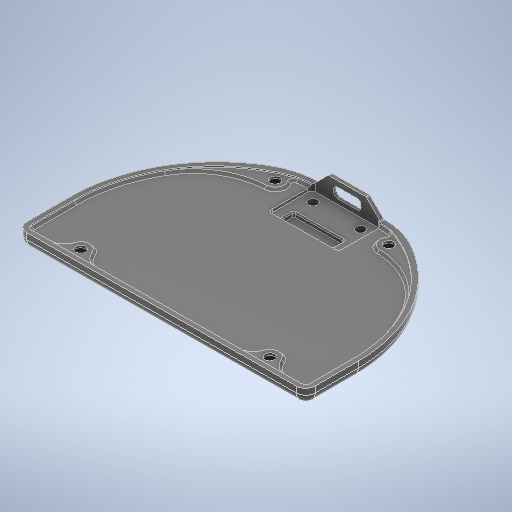
# Autodesk Inventor part: Bottom
Saved by Autodesk Inventor 2025.3 (Build 293356030, 356C)
## iProperties
Created: 2024-12-25
Part Number: Bottom
Material: Acetal Resin, Black
Document SubType Name: Modeling
Designer: tvoko
Density: 1.425 g/cm^3
Appearance: Smooth - Black
Author: tvoko
Autodesk Inventor part; units mm, degrees
ref_plane "YZ Plane" through (0, 0, 0) normal (1, 0, 0) x (0, 1, 0)
ref_plane "XZ Plane" through (0, 0, 0) normal (0, 1, 0) x (-1, 0, 0)
ref_plane "XY Plane" through (0, 0, 0) normal (0, 0, 1) x (1, 0, 0)
ref_plane "Work Plane1" through (11.8275, -6.9783, -10.6662) normal (0.0061942, -0.9999808, -0.0000034) x (0.9999802, 0.0061942, -0.0010922)
sketch "Sketch1" plane through (11.8275, -6.9783, -10.6662) normal (0.0061942, -0.9999808, -0.0000034) x (0.9999802, 0.0061942, -0.0010922)
  line L0 (-55.0975, -59.86) -> (-32.8725, -59.86)
  line L1 (-1.1225, 0.465) -> (-86.8475, 0.465)
  line L2 (-32.8725, -61.4475) -> (-55.0975, -61.4475)
  line L3 (-86.8475, 2.0525) -> (-1.1225, 2.0525)
  circle A0 centre (-24.935, -55.287) radius 1.6
  circle A1 centre (-63.035, -55.287) radius 1.6
  circle A2 centre (-75.735, -2.535) radius 1.6
  circle A3 centre (-12.235, -2.535) radius 1.6
  line L4 (-7.8704, 0.465) -> (-16.5997, 0.465)
  line L5 (-71.3704, 0.465) -> (-80.0997, 0.465)
  line L6 (-55.2619, -59.8595) -> (-55.2619, -61.447) projected
  arc A4 (-59.548, -59.4404) -> (-55.2619, -59.8595) centre (-55.0975, -36.0475) ccw projected
  arc A5 (-60.5607, -56.9833) -> (-59.548, -59.4404) centre (-59.2513, -57.8809) ccw projected
  arc A6 (-60.5607, -56.9833) -> (-62.9204, -52.2892) centre (-63.035, -55.287) ccw projected
  arc A7 (-84.3659, -39.412) -> (-62.9204, -52.2892) centre (-61.9279, -26.3401) ccw projected
  arc A8 (-90.8163, -15.5257) -> (-84.3659, -39.412) centre (-43.3648, -15.5257) ccw projected
  line L7 (-90.8163, -15.5257) -> (-90.8163, -1.1225) projected
  arc A9 (-89.2288, 0.465) -> (-90.8163, -1.1225) centre (-89.2288, -1.1225) ccw projected
  line L8 (-89.2288, 0.465) -> (-84.4643, 0.465) projected
  arc A10 (-78.5359, -3.6099) -> (-84.4643, 0.465) centre (-84.4643, -5.885) ccw projected
  arc A11 (-78.5359, -3.6099) -> (-72.9342, -3.6099) centre (-75.735, -2.535) ccw projected
  arc A12 (-67.0058, 0.465) -> (-72.9342, -3.6099) centre (-67.0058, -5.885) ccw projected
  line L9 (-67.0058, 0.465) -> (-20.9643, 0.465) projected
  arc A13 (-15.0359, -3.6099) -> (-20.9643, 0.465) centre (-20.9643, -5.885) ccw projected
  arc A14 (-15.0359, -3.6099) -> (-9.4342, -3.6099) centre (-12.235, -2.535) ccw projected
  arc A15 (-3.5058, 0.465) -> (-9.4342, -3.6099) centre (-3.5058, -5.885) ccw projected
  line L10 (-3.5058, 0.465) -> (1.2587, 0.465) projected
  arc A16 (2.8462, -1.1225) -> (1.2587, 0.465) centre (1.2587, -1.1225) ccw projected
  line L11 (2.8462, -1.1225) -> (2.8462, -15.5257) projected
  arc A17 (-3.6042, -39.412) -> (2.8462, -15.5257) centre (-44.6053, -15.5257) ccw projected
  arc A18 (-25.0497, -52.2892) -> (-3.6042, -39.412) centre (-26.0422, -26.3401) ccw projected
  arc A19 (-25.0497, -52.2892) -> (-27.4094, -56.9833) centre (-24.935, -55.287) ccw projected
  arc A20 (-28.4221, -59.4404) -> (-27.4094, -56.9833) centre (-28.7188, -57.8809) ccw projected
  arc A21 (-32.7081, -59.8595) -> (-28.4221, -59.4404) centre (-32.8725, -36.0475) ccw projected
  line L12 (-32.7081, -61.447) -> (-32.7081, -59.8595) projected
  arc A22 (-32.7081, -61.447) -> (-20.2658, -58.0981) centre (-32.8725, -36.0475) ccw projected
  arc A23 (-20.2658, -58.0981) -> (4.4337, -15.5257) centre (-44.6053, -15.5257) ccw projected
  line L13 (4.4337, -1.1225) -> (4.4337, -15.5257) projected
  arc A24 (4.4337, -1.1225) -> (1.2587, 2.0525) centre (1.2587, -1.1225) ccw projected
  line L14 (1.2587, 2.0525) -> (-89.2288, 2.0525) projected
  arc A25 (-89.2288, 2.0525) -> (-92.4038, -1.1225) centre (-89.2288, -1.1225) ccw projected
  line L15 (-92.4038, -15.5257) -> (-92.4038, -1.1225) projected
  arc A26 (-92.4038, -15.5257) -> (-67.7043, -58.0981) centre (-43.3648, -15.5257) ccw projected
  arc A27 (-67.7043, -58.0981) -> (-55.2619, -61.447) centre (-55.0975, -36.0475) ccw projected
  circle A28 centre (-12.235, -2.535) radius 1.5 projected
  circle A29 centre (-24.935, -55.287) radius 1.5 projected
  circle A30 centre (-75.735, -2.535) radius 1.5 projected
  circle A31 centre (-63.035, -55.287) radius 1.5 projected
  line L16 (-55.2619, -61.447) -> (-32.7081, -61.447)
  line L17 (-32.7081, -59.8595) -> (-55.2619, -59.8595)
  point P0 (-11.7957, 10.6533)
  point P1 (-88.435, -15.5257)
  point P2 (-70.4688, -54.2343)
  point P3 (-17.5013, -54.2343)
  point P4 (0.465, -15.5257)
  point P5 (0.465, -1.1225)
  point P6 (-88.435, -1.1225)
  point P7 (-71.4936, -55.4468)
  point P8 (-90.0225, -15.5257)
  point P9 (-90.0225, -1.1225)
  point P10 (2.0525, -1.1225)
  point P11 (2.0525, -15.5257)
  point P12 (-16.4765, -55.4468)
  dimension "d0" = 3.2
  constraints: 14 end point, 6 horizontal, 4 centre point, 4 coincident, 3 equal radius, 1 parallel, 1 point on circle, 23 other
  measures "d0" diameter of A0
extrude "Extrusion1" add sketch "Sketch1" along normal blind 1.1906 contours L0 L17 L12 L16 L2 L6 | L6 A27 A26 L15 A25 L14 L3 A24 L13 A23 A22 L12 A21 A20 A19 A18 A17 L11 A16 L10 L1 L8 A9 L7 A8 A7 A6 A5 A4 | L1 A12 A11 A10 | A15 A14 A13 L1
sketch "Sketch2" plane through (11.8349, -8.1689, -10.6662) normal (0.0061942, -0.9999808, -0.0000034) x (0.9999802, 0.0061942, -0.0010922)
  line L0 (1.2587, 2.0525) -> (-89.2288, 2.0525) projected
  circle A0 centre (-12.235, -2.535) radius 1.6 projected
  circle A1 centre (-24.935, -55.287) radius 1.6 projected
  circle A2 centre (-63.035, -55.287) radius 1.6 projected
  circle A3 centre (-75.735, -2.535) radius 1.6 projected
  circle A4 centre (-75.735, -2.535) radius 2.95
  circle A5 centre (-12.235, -2.535) radius 2.95
  circle A6 centre (-24.935, -55.287) radius 2.95
  circle A7 centre (-63.035, -55.287) radius 2.95
  arc A8 (-20.2658, -58.0981) -> (4.4337, -15.5257) centre (-44.6053, -15.5257) ccw projected
  line L1 (4.4337, -15.5257) -> (4.4337, -1.1225) projected
  arc A9 (4.4337, -1.1225) -> (1.2587, 2.0525) centre (1.2587, -1.1225) ccw projected
  line L2 (1.2587, 2.0525) -> (-89.2288, 2.0525) projected
  arc A10 (-89.2288, 2.0525) -> (-92.4038, -1.1225) centre (-89.2288, -1.1225) ccw projected
  line L3 (-92.4038, -1.1225) -> (-92.4038, -15.5257) projected
  arc A11 (-92.4038, -15.5257) -> (-67.7043, -58.0981) centre (-43.3648, -15.5257) ccw projected
  arc A12 (-67.7043, -58.0981) -> (-55.2619, -61.447) centre (-55.0975, -36.0475) ccw projected
  line L4 (-55.2619, -61.447) -> (-32.7081, -61.447) projected
  arc A13 (-32.7081, -61.447) -> (-20.2658, -58.0981) centre (-32.8725, -36.0475) ccw projected
  circle A14 centre (-75.735, -2.535) radius 1.6 projected
  circle A15 centre (-12.235, -2.535) radius 1.6 projected
  circle A16 centre (-63.035, -55.287) radius 1.6 projected
  circle A17 centre (-24.935, -55.287) radius 1.6 projected
  point P0 (-11.7957, 10.6533)
  point P1 (-24.935, -55.287)
  point P2 (-63.035, -55.287)
  point P3 (1.2587, 2.0525)
  point P4 (-89.2288, 2.0525)
  dimension "d4" = 5.9
  constraints: 4 centre point, 4 coincident, 3 equal radius
  measures "d4" diameter of A4
extrude "Extrusion2" add sketch "Sketch2" along normal blind 4 contours A9 L1 A8 A13 L4 A12 A11 L3 A10 L0
fillet "Fillet1" radius 3.175 2 edges at (-32.1223, -12.4413, -8.5657) (-32.1916, -12.4415, -72.0652)
chamfer "Chamfer1" distance 0.7937 angle 45 24 edges at (-75.0094, -8.7069, -10.1064) (-69.0316, -8.6698, -11.2299) (-63.9047, -8.6381, -16.1185) (-58.7671, -8.6062, -11.2411) (-32.1488, -8.4414, -10.1532) (-5.5329, -8.2765, -11.2992) (-0.406, -8.2447, -16.1879) (4.7316, -8.2129, -11.3104) (10.7119, -8.1759, -10.2) (14.2161, -8.1542, -10.6688) (14.6719, -8.1513, -18.9935) (13.0096, -8.1615, -38.5642) (-0.8922, -8.2476, -59.2553) (-15.8389, -8.3402, -64.5756) (-15.4795, -8.3379, -69.1222) (-18.7854, -8.3584, -70.3799) (-78.5146, -8.7286, -10.5675) (-78.9887, -8.7315, -18.8912) (-77.3691, -8.7214, -38.4655) (-63.5126, -8.6355, -59.1869) (-48.5775, -8.5429, -64.5398) (-48.9468, -8.5452, -69.0857) (-45.6437, -8.5248, -70.3505) (-32.2147, -8.4416, -70.4776)
sketch "Sketch3" plane through (11.8275, -6.9783, -10.6662) normal (-0.0061942, 0.9999808, 0.0000034) x (0.9999802, 0.0061942, -0.0010922)
  arc A0 (-20.2658, 58.0981) -> (-32.7081, 61.447) centre (-32.8725, 36.0475) ccw projected
  line L0 (-55.2619, 61.447) -> (-32.7081, 61.447) projected
  arc A1 (-55.2619, 61.447) -> (-67.7043, 58.0981) centre (-55.0975, 36.0475) ccw projected
  arc A2 (-67.7043, 58.0981) -> (-92.4038, 15.5257) centre (-43.3648, 15.5257) ccw projected
  line L1 (-92.4038, 1.1225) -> (-92.4038, 15.5257) projected
  arc A3 (-92.4038, 1.1225) -> (-89.2288, -2.0525) centre (-89.2288, 1.1225) ccw projected
  line L2 (1.2587, -2.0525) -> (-89.2288, -2.0525) projected
  arc A4 (1.2587, -2.0525) -> (4.4337, 1.1225) centre (1.2587, 1.1225) ccw projected
  line L3 (4.4337, 15.5257) -> (4.4337, 1.1225) projected
  arc A5 (4.4337, 15.5257) -> (-20.2658, 58.0981) centre (-44.6053, 15.5257) ccw projected
  arc A6 (-55.2619, 59.8595) -> (-59.548, 59.4404) centre (-55.0975, 36.0475) ccw projected
  line L4 (-32.7081, 59.8595) -> (-55.2619, 59.8595) projected
  arc A7 (-28.4221, 59.4404) -> (-32.7081, 59.8595) centre (-32.8725, 36.0475) ccw projected
  arc A8 (-27.4094, 56.9833) -> (-28.4221, 59.4404) centre (-28.7188, 57.8809) ccw projected
  arc A9 (-27.4094, 56.9833) -> (-25.0497, 52.2892) centre (-24.935, 55.287) ccw projected
  arc A10 (-3.6042, 39.412) -> (-25.0497, 52.2892) centre (-26.0422, 26.3401) ccw projected
  arc A11 (2.8462, 15.5257) -> (-3.6042, 39.412) centre (-44.6053, 15.5257) ccw projected
  line L5 (2.8462, 1.1225) -> (2.8462, 15.5257) projected
  arc A12 (1.2587, -0.465) -> (2.8462, 1.1225) centre (1.2587, 1.1225) ccw projected
  line L6 (-3.5058, -0.465) -> (1.2587, -0.465) projected
  arc A13 (-9.4342, 3.6099) -> (-3.5058, -0.465) centre (-3.5058, 5.885) ccw projected
  arc A14 (-9.4342, 3.6099) -> (-15.0359, 3.6099) centre (-12.235, 2.535) ccw projected
  arc A15 (-20.9643, -0.465) -> (-15.0359, 3.6099) centre (-20.9643, 5.885) ccw projected
  line L7 (-67.0058, -0.465) -> (-20.9643, -0.465) projected
  arc A16 (-72.9342, 3.6099) -> (-67.0058, -0.465) centre (-67.0058, 5.885) ccw projected
  arc A17 (-72.9342, 3.6099) -> (-78.5359, 3.6099) centre (-75.735, 2.535) ccw projected
  arc A18 (-84.4643, -0.465) -> (-78.5359, 3.6099) centre (-84.4643, 5.885) ccw projected
  line L8 (-89.2288, -0.465) -> (-84.4643, -0.465) projected
  arc A19 (-90.8163, 1.1225) -> (-89.2288, -0.465) centre (-89.2288, 1.1225) ccw projected
  line L9 (-90.8163, 15.5257) -> (-90.8163, 1.1225) projected
  arc A20 (-84.3659, 39.412) -> (-90.8163, 15.5257) centre (-43.3648, 15.5257) ccw projected
  arc A21 (-62.9204, 52.2892) -> (-84.3659, 39.412) centre (-61.9279, 26.3401) ccw projected
  arc A22 (-62.9204, 52.2892) -> (-60.5607, 56.9833) centre (-63.035, 55.287) ccw projected
  arc A23 (-59.548, 59.4404) -> (-60.5607, 56.9833) centre (-59.2513, 57.8809) ccw projected
  circle A24 centre (-75.735, 2.535) radius 1.6 projected
  circle A25 centre (-24.935, 55.287) radius 1.6 projected
  circle A26 centre (-63.035, 55.287) radius 1.6 projected
  circle A27 centre (-12.235, 2.535) radius 1.6 projected
  line L10 (-84.4643, -0.465) -> (-67.0058, -0.465)
  arc A28 (-84.4643, -0.465) -> (-78.5359, 3.6099) centre (-84.4643, 5.885) ccw projected
  line L11 (-20.9643, -0.465) -> (-3.5058, -0.465)
  arc A29 (-59.7509, 59.3877) -> (-84.3659, 39.412) centre (-45.648, 16.8559) ccw
  arc A30 (-62.9204, 52.2892) -> (-84.3659, 39.412) centre (-61.9279, 26.3401) ccw projected
  arc A31 (-59.548, 59.4404) -> (-60.5607, 56.9833) centre (-59.2513, 57.8809) ccw projected
  arc A32 (-3.6042, 39.412) -> (-28.2191, 59.3877) centre (-42.3221, 16.8559) ccw
  arc A33 (-3.6042, 39.412) -> (-25.0497, 52.2892) centre (-26.0422, 26.3401) ccw projected
  point P0 (-59.7509, 59.3877)
  constraints: 7 tangent, 6 point on circle, 4 end point, 2 centre point, 1 collinear, 1 horizontal
extrude "Extrusion3" cut sketch "Sketch3" against normal blind 0.3969 contours A23 A22 A21 A29 | A32 A10 A9 A8 | A18 A17 A16 L10 | L11 A15 A14 A13
sketch "Sketch4" plane through (11.8349, -8.1689, -10.6662) normal (-0.0061942, 0.9999808, 0.0000034) x (0.9999802, 0.0061942, -0.0010922)
  line L0 (-84.4643, 0.3288) -> (-89.2288, 0.3288) projected
  line L1 (-43.985, 59.0646) -> (-43.985, 0.3288) construction
  line L2 (-35.985, 56.8657) -> (-51.985, 56.8657) construction
  line L3 (-51.985, 56.8657) -> (-35.985, 56.8657) construction
  circle A0 centre (-51.985, 56.8657) radius 1.5
  circle A1 centre (-35.985, 56.8657) radius 1.5
  line L4 (-33.485, 46.4657) -> (-54.485, 46.4657) construction
  line L5 (-54.985, 46.9657) -> (-54.985, 58.9657) construction
  line L6 (-54.485, 59.4657) -> (-33.485, 59.4657) construction
  line L7 (-32.985, 58.9657) -> (-32.985, 46.9657) construction
  arc A2 (-33.485, 46.4657) -> (-32.985, 46.9657) centre (-33.485, 46.9657) ccw construction
  arc A3 (-54.985, 46.9657) -> (-54.485, 46.4657) centre (-54.485, 46.9657) ccw construction
  arc A4 (-54.485, 59.4657) -> (-54.985, 58.9657) centre (-54.485, 58.9657) ccw construction
  arc A5 (-32.985, 58.9657) -> (-33.485, 59.4657) centre (-33.485, 58.9657) ccw construction
  line L8 (-55.785, 58.9657) -> (-55.785, 46.9657)
  arc A6 (-55.785, 46.9657) -> (-54.485, 45.6657) centre (-54.485, 46.9657) ccw
  line L9 (-54.485, 45.6657) -> (-33.485, 45.6657)
  arc A7 (-33.485, 45.6657) -> (-32.185, 46.9657) centre (-33.485, 46.9657) ccw
  line L10 (-32.185, 46.9657) -> (-32.185, 58.9657)
  arc A8 (-32.185, 58.9657) -> (-33.485, 60.2657) centre (-33.485, 58.9657) ccw
  line L11 (-33.485, 60.2657) -> (-54.485, 60.2657)
  arc A9 (-54.485, 60.2657) -> (-55.785, 58.9657) centre (-54.485, 58.9657) ccw
  line L12 (-51.985, 56.8657) -> (-51.985, 55.3657) construction
  line L13 (-51.985, 50.8657) -> (-35.985, 50.8657)
  line L14 (-35.485, 50.3657) -> (-35.485, 47.3657)
  line L15 (-35.985, 46.8657) -> (-51.985, 46.8657)
  line L16 (-52.485, 47.3657) -> (-52.485, 50.3657)
  arc A10 (-51.985, 50.8657) -> (-52.485, 50.3657) centre (-51.985, 50.3657) ccw
  arc A11 (-52.485, 47.3657) -> (-51.985, 46.8657) centre (-51.985, 47.3657) ccw
  arc A12 (-35.985, 46.8657) -> (-35.485, 47.3657) centre (-35.985, 47.3657) ccw
  arc A13 (-35.485, 50.3657) -> (-35.985, 50.8657) centre (-35.985, 50.3657) ccw
  line L17 (-55.685, 59.4657) -> (-32.285, 59.4657)
  line L18 (-55.2592, 59.0657) -> (-32.7109, 59.0657) projected
  arc A14 (-55.2592, 59.0657) -> (-59.3997, 58.6607) centre (-55.0975, 36.0475) ccw projected
  arc A15 (-59.3997, 58.6607) -> (-59.906, 57.4321) centre (-59.2513, 57.8809) ccw projected
  arc A16 (-62.89, 51.496) -> (-59.906, 57.4321) centre (-63.035, 55.287) ccw projected
  arc A17 (-62.89, 51.496) -> (-83.6801, 39.0124) centre (-61.9279, 26.3401) ccw projected
  arc A18 (-83.6801, 39.0124) -> (-90.0225, 15.5257) centre (-43.3648, 15.5257) ccw projected
  line L19 (-90.0225, 1.1225) -> (-90.0225, 15.5257) projected
  arc A19 (-90.0225, 1.1225) -> (-89.2288, 0.3288) centre (-89.2288, 1.1225) ccw projected
  arc A20 (-84.4643, 0.3288) -> (-79.2769, 3.8943) centre (-84.4643, 5.885) ccw projected
  arc A21 (-72.1931, 3.8943) -> (-79.2769, 3.8943) centre (-75.735, 2.535) ccw projected
  arc A22 (-72.1931, 3.8943) -> (-67.0058, 0.3288) centre (-67.0058, 5.885) ccw projected
  line L20 (-20.9643, 0.3288) -> (-67.0058, 0.3288) projected
  arc A23 (-20.9643, 0.3288) -> (-15.7769, 3.8943) centre (-20.9643, 5.885) ccw projected
  arc A24 (-8.6931, 3.8943) -> (-15.7769, 3.8943) centre (-12.235, 2.535) ccw projected
  arc A25 (-8.6931, 3.8943) -> (-3.5058, 0.3288) centre (-3.5058, 5.885) ccw projected
  line L21 (1.2587, 0.3288) -> (-3.5058, 0.3288) projected
  arc A26 (1.2587, 0.3288) -> (2.0525, 1.1225) centre (1.2587, 1.1225) ccw projected
  line L22 (2.0525, 15.5257) -> (2.0525, 1.1225) projected
  arc A27 (2.0525, 15.5257) -> (-4.29, 39.0124) centre (-44.6053, 15.5257) ccw projected
  arc A28 (-4.29, 39.0124) -> (-25.08, 51.496) centre (-26.0422, 26.3401) ccw projected
  arc A29 (-28.0641, 57.4321) -> (-25.08, 51.496) centre (-24.935, 55.287) ccw projected
  arc A30 (-28.0641, 57.4321) -> (-28.5704, 58.6607) centre (-28.7188, 57.8809) ccw projected
  arc A31 (-28.5704, 58.6607) -> (-32.7109, 59.0657) centre (-32.8725, 36.0475) ccw projected
  point P0 (-11.7957, -10.6533)
  point P1 (-52.485, 46.8657)
  point P2 (-43.985, 50.8657)
  point P3 (-43.985, 46.4657)
  point P4 (-43.985, 56.8657)
  point P5 (-43.985, 56.8657)
  dimension "d55" = 3
  dimension "d22" = 16
  dimension "d24" = 22
  dimension "d26" = 2.6
  dimension "d28" = 0.5
  dimension "d57" = 0.8
  dimension "d59" = 4
  dimension "d60" = 17
  dimension "d62" = 0.5
  dimension "d63" = 13
  dimension "d68" = 6
  dimension "d75" = 2.2
  constraints: 34 end point, 26 point on circle, 16 tangent, 13 centre point, 8 point on line, 7 equal length, 6 equal radius, 5 midpoint, 4 perpendicular, 3 horizontal, 2 coincident, 1 vertical, 1 vertical alignment, 10 other
  measures "d22" distance of L2.end L3.end
  measures "d24" distance between parallel lines of L7 L5
  measures "d26" distance from line of L6 L3.end
  measures "d28" radius of A2
  measures "d57" distance between parallel lines of L7 L10
  measures "d59" distance between parallel lines of L15 L13
  measures "d60" distance between parallel lines of L14 L16
  measures "d62" radius of A10
  measures "d63" distance between parallel lines of L6 L4
  measures "d68" distance between parallel lines of L2 L13
  measures "d75" distance between parallel lines of L18 L2
extrude "Extrusion4" cut sketch "Sketch4" against normal blind 3 contours A0 | A1
extrude "Extrusion6" cut sketch "Sketch4" against normal blind 1 contours A14 L18 A31 A8 L10 A7 L9 A6 L8 A9 | A9 L17 A8 A31 L18 A14 | A9 L11 A8 L17 | A0 | A1 | L13 A13 L14 A12 L15 A11 L16 A10
extrude "Extrusion7" cut sketch "Sketch4" along normal through all contours A14 L18 A31 A8 L10 A7 L9 A6 L8 A9 | A9 L17 A8 A31 L18 A14 | A9 L11 A8 L17 | A0 | A1 | L13 A13 L14 A12 L15 A11 L16 A10
sketch "Sketch5" plane through (-21.1115, -7.1821, -72.0773) normal (-0.0010922, -0.0000034, -0.9999994) x (-0.9999802, -0.0061942, 0.0010922)
  line L0 (22.3894, 0) -> (-0.4932, 0)
  line L1 (10.9481, 0) -> (10.9481, 4.7625) construction
  line L2 (4.5981, 4.7625) -> (17.2981, 4.7625)
  line L3 (17.2981, 4.7625) -> (22.0606, 0)
  line L4 (4.5981, 4.7625) -> (-0.1644, 0)
  line L5 (6.4481, 1.5125) -> (6.4481, 0.8525)
  arc A0 (6.4481, 0.8525) -> (7.6981, -0.3975) centre (7.6981, 0.8525) ccw
  line L6 (7.6981, -0.3975) -> (14.1981, -0.3975)
  arc A1 (14.1981, -0.3975) -> (15.4481, 0.8525) centre (14.1981, 0.8525) ccw
  line L7 (15.4481, 0.8525) -> (15.4481, 1.5125)
  arc A2 (15.4481, 1.5125) -> (14.1981, 2.7625) centre (14.1981, 1.5125) ccw
  line L8 (14.1981, 2.7625) -> (7.6981, 2.7625)
  arc A3 (7.6981, 2.7625) -> (6.4481, 1.5125) centre (7.6981, 1.5125) ccw
  line L9 (6.3481, 1.5125) -> (6.3481, 0.8525)
  arc A4 (6.3481, 0.8525) -> (7.6981, -0.4975) centre (7.6981, 0.8525) ccw
  line L10 (7.6981, -0.4975) -> (14.1981, -0.4975)
  arc A5 (14.1981, -0.4975) -> (15.5481, 0.8525) centre (14.1981, 0.8525) ccw
  line L11 (15.5481, 0.8525) -> (15.5481, 1.5125)
  arc A6 (15.5481, 1.5125) -> (14.1981, 2.8625) centre (14.1981, 1.5125) ccw
  line L12 (14.1981, 2.8625) -> (7.6981, 2.8625)
  arc A7 (7.6981, 2.8625) -> (6.3481, 1.5125) centre (7.6981, 1.5125) ccw
  line L13 (22.3894, 0) -> (-0.1644, 0) projected
  point P0 (-21.0768, 7.0515)
  point P1 (10.9481, 2.7625)
  dimension "d33" = 45
  dimension "d34" = 12.7
  dimension "d35" = 4.7625
  dimension "d38" = 0.1
  dimension "d71" = 9
  dimension "d72" = 3.16
  dimension "d73" = 1.25
  dimension "d74" = 2
  constraints: 26 end point, 16 point on circle, 8 centre point, 8 tangent, 5 perpendicular, 3 equal radius, 3 midpoint, 3 point on line, 1 horizontal, 1 vertical, 7 other
  measures "d33" angle of L0 L4
  measures "d34" distance of L2.start L2.end
  measures "d35" distance of L1.start L1.end
  measures "d38" radial gap between concentric circles of A3 A7
  measures "d71" distance between parallel lines of L7 L5
  measures "d72" distance between parallel lines of L6 L8
  measures "d73" radius of A3
  measures "d74" distance between parallel lines of L2 L8
extrude "Extrusion8" add sketch "Sketch5" against normal up to surface (1.1813 mm away) contours L0 A5 L11 A6 L12 A7 L9 A4 L4 L2 L3 | L0 A1 L7 A2 L8 A3 L5 A0 A4 L9 A7 L12 A6 L11 A5 | L0 A0 L5 A3 L8 A2 L7 A1
fillet "Fillet3" radius 0.3969 4 edges at (-38.4381, -2.5269, -71.4677) (-25.7384, -2.4482, -71.4816) (-20.9465, -7.1811, -71.4868) (-43.171, -7.3188, -71.4625)
extrude "Extrusion10" cut sketch "Sketch4" against normal blind 2.5 contours L13 A13 L14 A12 L15 A11 L16 A10
fillet "Fillet4" radius 0.3969 8 edges at (-23.8451, -9.3918, -61.3465) (-23.6966, -9.3909, -59.4932) (-23.841, -9.3918, -57.6394) (-32.1943, -9.4435, -57.4839) (-40.5478, -9.4953, -57.6212) (-40.6963, -9.4962, -59.4746) (-40.5519, -9.4953, -61.3283) (-32.1986, -9.4435, -61.4839)
extrude "Extrusion11" cut sketch "Sketch5" against normal blind 2 contours A5 L10 A4 L0 A0 L6 A1 | L0 A1 L7 A2 L8 A3 L5 A0 A4 L9 A7 L12 A6 L11 A5 | A1 L6 A0 L0 | L0 A0 L5 A3 L8 A2 L7 A1
fillet "Fillet5" radius 0.5 8 edges at (-27.4668, -6.039, -72.0703) (-27.8702, -4.7569, -72.0699) (-32.0771, -4.3875, -72.0653) (-36.2792, -4.809, -72.0607) (-36.6666, -6.096, -72.0603) (-36.2633, -7.3781, -72.0607) (-32.0563, -7.7474, -72.0653) (-27.8542, -7.326, -72.0699)
body "Solid1"
